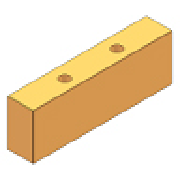
# Autodesk Inventor part: SA-SB-400x400x90
Saved by Autodesk Inventor 2024 (Build 280153000, 153)
## iProperties
Created: 2023-01-19
Part Number: SA-SB-400x400x90
Material: S 55 C
Description: Spacer Block
Document SubType Name: Modeling
Designer: Alex
Standard Revision: 1
Manufacturer: FUTABA
Language: en-US
Size Designation: 400x400x90
Categories: <MemberInstance><Categories><Category DisplayName="Mold" InternalName="349578f2-f4d4-4954-8c09-8e99297a61c0" Mnemonic="MOLD"><Category DisplayName="Mold Plates" InternalName="034241f0-2fc6-4170-ab7c-5d11f2fd1ecc" Mnemonic="MOLD PLATES"><Category DisplayName="Spacer Blocks" InternalName="a8712dcd-2322-49ba-a5db-da2c8d28e342" Mnemonic="SPACER BLOCKS"><CategoryParameter DisplayName="Plate Width" InternalName="193016f8-b965-48fc-ab20-dcb8e737aa26" Mnemonic="PLATE WIDTH"/><CategoryParameter DisplayName="Plate Property" InternalName="19950201-27b9-4c21-8f8e-d51abcbf9294" Mnemonic="PLATE PROPERTY"/><CategoryParameter DisplayName="Plate Height" InternalName="25512d79-b911-4596-9cd9-933d6fa548d9" Mnemonic="PLATE HEIGTH"/><CategoryParameter DisplayName="Mold Base Length" InternalName="2d45cff1-b12d-4425-b864-6391a393b446" Mnemonic="MOLD BASE LENGTH"/><CategoryParameter DisplayName="Plate Position" InternalName="8806bcf5-3ca1-4d27-9110-78cdfbd806d6" Mnemonic="PLATE POSITION"/><CategoryParameter DisplayName="Mold Base Width" InternalName="ad8184d4-fe16-432a-a315-a30dcf6563a0" Mnemonic="MOLD BASE WIDTH"/><CategoryParameter DisplayName="Interval Width" InternalName="b2b42416-4aca-44bf-8951-b37bc3b2cbd3" Mnemonic="INTERVAL WIDTH"/><CategoryParameter DisplayName="Plate Number" InternalName="d678c198-6967-4c5a-9ee9-53f54c0eeff5" Mnemonic="PLATE NUMBER"/><Category DisplayName="LR" InternalName="6b8a849a-1520-47a0-b375-241d54a05680" Mnemonic="LR"/></Category></Category></Category><Category DisplayName="DataType" InternalName="23b78d0f-2648-40c6-8793-ca6db495c9e8" Mnemonic="DATATYPE"><CategoryParameter DisplayName="DisplayName" InternalName="05415f3d-3907-474b-a020-eb9d644f4cf3" Mnemonic="DISPLAYNAME"/><CategoryParameter DisplayName="Standard" InternalName="0c0a119c-1e12-4c84-803f-101930972f5e" Mnemonic="STANDARD"/><CategoryParameter DisplayName="Description" InternalName="13903e3d-64b1-4950-80da-f627842ea37f" Mnemonic="DESCRIPTION"/><CategoryParameter DisplayName="Designation" InternalName="2675968c-4ce5-49e0-a4f5-552d29089031" Mnemonic="DESIGNATION"/><CategoryParameter DisplayName="Default Row" InternalName="2af9ec52-faaa-4026-b378-f9fa4afca842" Mnemonic="DEFAULTROW"/><CategoryParameter DisplayName="Folder Name" InternalName="3f06958e-8713-4116-9be7-ed6184ecc97b" Mnemonic="FOLDERNAME"/><CategoryParameter DisplayName="Revision Guid" InternalName="45a75005-10b1-4dfc-8d6d-dfe629f0b93c" Mnemonic="REVISIONGUID"/><CategoryParameter DisplayName="FileName" InternalName="8b46a4cc-9585-4fed-90c3-899f57e09a73" Mnemonic="FILENAME"/><CategoryParameter DisplayName="StdsOrg" InternalName="8f5914e1-4693-403f-8ab5-d37768198c9d" Mnemonic="STDSORG"/><CategoryParameter DisplayName="Family Version" InternalName="914462f6-6e19-4b14-ba84-155b9680b1d0" Mnemonic="FAMILYREVISION"/><CategoryParameter DisplayName="Standard Revision" InternalName="91d5a463-65c2-4fde-b823-3b7fea5e8e17" Mnemonic="STANDARDREVISION"/><CategoryParameter DisplayName="Member Revision" InternalName="a65d44b9-392f-4f4f-857b-e4b3d54996fe" Mnemonic="MEMBERREVISION"/><CategoryParameter DisplayName="ClipFormat" InternalName="bc51e27b-3422-4e78-93ef-cec197ddf230" Mnemonic="CLIPFORMAT"/><CategoryParameter DisplayName="Manufacturer" InternalName="cd6c7a72-a28a-4e50-99a9-2c7f4e13e5ad" Mnemonic="MANUFACTURER"/><CategoryParameter DisplayName="InternalName" InternalName="cf1d0246-76d9-4b4a-8305-fa0409afb5c1" Mnemonic="INTERNALNAME"/><CategoryParameter DisplayName="IsMetric" InternalName="e2385c5b-1ea4-4823-96a8-8de651266ec3" Mnemonic="ISMETRIC"/><Category DisplayName="Part" InternalName="c0e0b642-3bcb-4cc8-9e80-f96d35c4afa4" Mnemonic="PART"><CategoryParameter DisplayName="Part Number" InternalName="016b6077-bfbe-49bd-92c9-d8d59c39c941" Mnemonic="PARTNUMBER"/><CategoryParameter DisplayName="Stock Number" InternalName="4dba7c1c-e26c-444e-836c-b08b433409a8" Mnemonic="STOCKNUMBER"/><CategoryParameter DisplayName="Material Key" InternalName="5c9a8adb-dd2b-4535-b97f-0a94a95fe41f" Mnemonic="MATERIALKEY"/><CategoryParameter DisplayName="Material" InternalName="818a152a-d3c3-49ca-80ee-df7d91421b8e" Mnemonic="MATERIAL"/></Category></Category></Categories><FamilyTemplate Id="SA-SB"><FamilyTemplateParameters><FamilyTemplateParameter ObjectType="kUserParameterObject" ValueType="xs:double" Id="1" ObjectReferenceKey="L"/><FamilyTemplateParameter ObjectType="kUserParameterObject" ValueType="xs:double" Id="2" ObjectReferenceKey="W_"/><FamilyTemplateParameter ObjectType="kUserParameterObject" ValueType="xs:double" Id="3" ObjectReferenceKey="H_"/><FamilyTemplateParameter ObjectType="kUserParameterObject" ValueType="xs:double" Id="4" ObjectReferenceKey="M_W"/><FamilyTemplateParameter ObjectType="kUserParameterObject" ValueType="xs:double" Id="5" ObjectReferenceKey="S1_L"/><FamilyTemplateParameter ObjectType="kUserParameterObject" ValueType="xs:double" Id="6" ObjectReferenceKey="S1_W"/><FamilyTemplateParameter ObjectType="kUserParameterObject" ValueType="xs:double" Id="7" ObjectReferenceKey="S1_d1"/><FamilyTemplateParameter ObjectType="kUserParameterObject" ValueType="xs:double" Id="8" ObjectReferenceKey="Ns"/><FamilyTemplateParameter ObjectType="kPartFeatureObject" ValueType="xs:boolean" Id="9" ObjectReferenceKey="1002000010000000aa010000000000008000000000000000" SubObjectId="Suppressed"/><FamilyTemplateParameter ObjectType="kPartFeatureObject" ValueType="xs:boolean" Id="10" ObjectReferenceKey="10020000100000006a360000000000008000000000000000" SubObjectId="Suppressed"/><FamilyTemplateParameter ObjectType="kPartComponentDefinitionObject" ValueType="xs:string" Id="11" SubObjectId="Material"/><FamilyTemplateParameter ObjectType="kPropertyObject" ValueType="xs:string" Id="20" ObjectReferenceKey="{32853F0F-3444-11d1-9E93-0060B03C1CA6}" SubObjectId="5"/><FamilyTemplateParameter ObjectType="kPropertyObject" ValueType="xs:string" Id="21" ObjectReferenceKey="{32853F0F-3444-11d1-9E93-0060B03C1CA6}" SubObjectId="52"/></FamilyTemplateParameters></FamilyTemplate><CategoryParameterMap><ParamToTemplateMap><ParamToTemplate CategoryParameter="//CategoryParameter[@InternalName='2af9ec52-faaa-4026-b378-f9fa4afca842']" ConstantValue="1"/><ParamToTemplate CategoryParameter="//CategoryParameter[@InternalName='bc51e27b-3422-4e78-93ef-cec197ddf230']" ConstantValue="CF_INVENTOR.STDPARTS"/><ParamToTemplate CategoryParameter="//CategoryParameter[@InternalName='e2385c5b-1ea4-4823-96a8-8de651266ec3']" ConstantValue="true"/><ParamToTemplate CategoryParameter="//CategoryParameter[@InternalName='cf1d0246-76d9-4b4a-8305-fa0409afb5c1']" ConstantValue="f32d549e-4bfe-4fe5-894e-412cfa612952"/><ParamToTemplate CategoryParameter="//CategoryParameter[@InternalName='45a75005-10b1-4dfc-8d6d-dfe629f0b93c']" ConstantValue="bfd3e5bc-12b0-4727-9f3c-e13b2a7c49ae"/><ParamToTemplate CategoryParameter="//CategoryParameter[@InternalName='3f06958e-8713-4116-9be7-ed6184ecc97b']" ConstantValue="SA-SB"/><ParamToTemplate CategoryParameter="//CategoryParameter[@InternalName='8f5914e1-4693-403f-8ab5-d37768198c9d']" TemplateParameter="15"/><ParamToTemplate CategoryParameter="//CategoryParameter[@InternalName='0c0a119c-1e12-4c84-803f-101930972f5e']" TemplateParameter="16"/><ParamToTemplate CategoryParameter="//CategoryParameter[@InternalName='91d5a463-65c2-4fde-b823-3b7fea5e8e17']" ConstantValue="1"/><ParamToTemplate CategoryParameter="//CategoryParameter[@InternalName='cd6c7a72-a28a-4e50-99a9-2c7f4e13e5ad']" ConstantValue="FUTABA"/><ParamToTemplate CategoryParameter="//CategoryParameter[@InternalName='13903e3d-64b1-4950-80da-f627842ea37f']" ConstantValue="Spacer Block"/><ParamToTemplate CategoryParameter="//CategoryParameter[@InternalName='05415f3d-3907-474b-a020-eb9d644f4cf3']" ConstantValue="SA-SB"/><ParamToTemplate CategoryParameter="//CategoryParameter[@InternalName='914462f6-6e19-4b14-ba84-155b9680b1d0']" ConstantValue="1"/><ParamToTemplate CategoryParameter="//CategoryParameter[@InternalName='bc51e27b-3422-4e78-93ef-cec197ddf230']" ConstantValue="CF_INVENTOR.STDPARTS"/><ParamToTemplate CategoryParameter="//CategoryParameter[@InternalName='8b46a4cc-9585-4fed-90c3-899f57e09a73']" ConstantValue="SA-SB-400x400x90"/><ParamToTemplate CategoryParameter="//CategoryParameter[@InternalName='a65d44b9-392f-4f4f-857b-e4b3d54996fe']" ConstantValue="43051CFB-8214-40DD-8585-8956856BFB98"/><ParamToTemplate CategoryParameter="//CategoryParameter[@InternalName='19950201-27b9-4c21-8f8e-d51abcbf9294']" ConstantValue="Spacer Block"/><ParamToTemplate CategoryParameter="//CategoryParameter[@InternalName='8806bcf5-3ca1-4d27-9110-78cdfbd806d6']" ConstantValue="L"/><ParamToTemplate CategoryParameter="//CategoryParameter[@InternalName='d678c198-6967-4c5a-9ee9-53f54c0eeff5']" ConstantValue="2"/><ParamToTemplate CategoryParameter="//CategoryParameter[@InternalName='2675968c-4ce5-49e0-a4f5-552d29089031']" TemplateParameter="21"/><ParamToTemplate CategoryParameter="//CategoryParameter[@InternalName='25512d79-b911-4596-9cd9-933d6fa548d9']" TemplateParameter="3"/><ParamToTemplate CategoryParameter="//CategoryParameter[@InternalName='2d45cff1-b12d-4425-b864-6391a393b446']" TemplateParameter="1"/><ParamToTemplate CategoryParameter="//CategoryParameter[@InternalName='818a152a-d3c3-49ca-80ee-df7d91421b8e']" TemplateParameter="11"/><ParamToTemplate CategoryParameter="//CategoryParameter[@InternalName='ad8184d4-fe16-432a-a315-a30dcf6563a0']" TemplateParameter="4"/><ParamToTemplate CategoryParameter="//CategoryParameter[@InternalName='016b6077-bfbe-49bd-92c9-d8d59c39c941']" TemplateParameter="20"/><ParamToTemplate CategoryParameter="//CategoryParameter[@InternalName='193016f8-b965-48fc-ab20-dcb8e737aa26']" TemplateParameter="2"/></ParamToTemplateMap></CategoryParameterMap></MemberInstance>
Density: 7.85 g/cm^3
Appearance: Orange (Pale)
IsCustomPart: 1
Author: Alex
Autodesk Inventor part; units mm, degrees
ref_plane "YZ Plane" through (0, 0, 0) normal (1, 0, 0) x (0, 1, 0)
sketch "Sketch1" plane through (0, 0, 0) normal (0, 0, 1) x (1, 0, 0)
  line L0 (-132, 200) -> (-200, 200)
  line L1 (-200, 200) -> (-200, -200)
  line L2 (-200, -200) -> (-132, -200)
  line L3 (-132, -200) -> (-132, 200)
  line L4 (200, 200) -> (200, -200)
  line L5 (132, -200) -> (132, 200)
  line L6 (132, 200) -> (200, 200)
  line L7 (132, -200) -> (200, -200)
  point P0 (0, 0)
  point P1 (-132, 0)
  point P2 (132, 0)
  point P3 (-165, 104)
  point P4 (165, 104)
  dimension "d85" = 400
  dimension "d86" = 68
  dimension "d88" = 68
  dimension "d89" = 200
  dimension "d93" = 400
  dimension "d94" = 200
  dimension "d98" = 104
  dimension "d100" = 165
  dimension "d101" = 165
  dimension "d102" = 104
  constraints: 16 end point, 3 parallel, 2 horizontal alignment, 2 midpoint, 2 perpendicular, 1 horizontal, 1 vertical
  measures "d85" distance between parallel lines of L2 L0
  measures "d86" distance between parallel lines of L3 L1
  measures "d88" distance between parallel lines of L4 L5
  measures "d89" distance from line of point (0, 0) L1
  measures "d93" distance between parallel lines of L7 L6
  measures "d94" distance from line of point (0, 0) L4
  measures "d98" vertical distance of point (-165, 104) point (0, 0)
  measures "d100" horizontal distance of point (-165, 104) point (0, 0)
  measures "d101" horizontal distance of point (165, 104) point (0, 0)
  measures "d102" vertical distance of point (0, 0) point (165, 104)
extrude "Extrusion1" [suppressed]
extrude "Extrusion2" add sketch "Sketch1" along normal blind 90 contours L4 L7 L5 L6
hole "Hole1" [suppressed]
pattern_linear "Rectangular Pattern1" [suppressed]
hole "Hole2" at (165, 104, 0) direction (0, 0, 1) diameter 18 depth 90
pattern_linear "Rectangular Pattern2" count 3 spacing 104 along (0, -1, 0) of "Hole2"
ref_plane "Work Plane1" through (0, 0, 90) normal (0, 0, 1) x (1, 0, 0)
ref_plane "Work Plane2" through (0, 0, 0) normal (0, 0, -1) x (-1, 0, 0)
chamfer "Chamfer1" [suppressed]
chamfer "Chamfer2" distance 0.5 angle 45 12 edges at (132, 0, 90) (200, 0, 90) (166, -200, 90) (132, -200, 45) (200, -200, 45) (166, -200, 0) (200, 0, 0) (132, 0, 0) (200, 200, 45) (166, 200, 90) (132, 200, 45) (166, 200, 0)
equation "\"d85\" = L"
equation "\"d86\" = W_"
equation "\"d88\" = W_"
equation "\"d89\" = 0.5 * M_W"
equation "\"d93\" = L"
equation "\"d94\" = 0.5 * M_W"
equation "\"d98\" = 0.5 * S1_L"
equation "\"d100\" = 0.5 * S1_W"
equation "\"d101\" = 0.5 * S1_W"
equation "\"d102\" = 0.5 * S1_L"
equation "\"d20\" = H_"
equation "\"d95\" = H_"
equation "\"d129\" = S1_d1"
equation "\"d134\" = H_"
equation "\"d122\" = S1_d1"
equation "\"d127\" = H_"
equation "\"L\" = 400"
equation "\"W_\" = 68"
equation "\"H_\" = 90"
equation "\"S1_d1\" = 18"
equation "\"M_W\" = 400"
equation "\"S1_L\" = 208"
equation "\"S1_W\" = 330"
body "Solid1"
